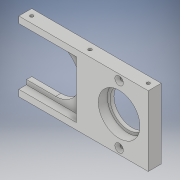
# Autodesk Inventor part: крепление подшипникового блока левая часть
Saved by Autodesk Inventor 2019.1 (Build 231200000, 200)
## iProperties
Created: 2018-08-01
Part Number: крепление подшипникового блока левая часть
Material: Типовые
Document SubType Name: Modeling
Designer: olege
Density: 1 g/cm^3
Appearance: По умолчанию
Author: olege
Autodesk Inventor part; units mm, degrees
ref_plane "YZ Plane" through (0, 0, 0) normal (1, 0, 0) x (0, 1, 0)
ref_plane "XZ Plane" through (0, 0, 0) normal (0, 1, 0) x (-1, 0, 0)
ref_plane "XY Plane" through (0, 0, 0) normal (0, 0, 1) x (1, 0, 0)
sketch "Эскиз1" plane through (0, 0, 0) normal (0, 0, 1) x (1, 0, 0)
  line L0 (50, -27) -> (-50, -27)
  line L1 (-50, -27) -> (-50, 27)
  line L2 (-50, 27) -> (50, 27)
  line L3 (50, 27) -> (50, -27)
  line L4 (50, -27) -> (-50, 27) construction
  line L5 (-50, -27) -> (50, 27) construction
  circle A0 centre (27.5, 0) radius 16.1
  point P0 (0, 0)
  point P1 (0, 0)
  dimension "d0" = 100
  dimension "d1" = 54
  dimension "d2" = 32.2
  dimension "d3" = 22.5
  constraints: 12 end point, 3 midpoint, 2 parallel, 1 centre point, 1 horizontal, 1 horizontal alignment, 1 perpendicular
  measures "d0" distance of L1.end L2.end
  measures "d1" distance of L0.end L1.end
  measures "d2" diameter of A0
  measures "d3" distance from line of L3 A0.centre
extrude "Выдавливание1" add sketch "Эскиз1" along normal blind 10
sketch "Эскиз2" plane through (0, 0, 0) normal (0, 0, -1) x (-1, 0, 0)
  circle A0 centre (-27.5, 0) radius 16.1 projected
  circle A1 centre (-27.5, 0) radius 14
  point P0 (0, 0)
  dimension "d6" = 28
  constraints: 1 centre point, 1 coincident
  measures "d6" diameter of A1
extrude "Выдавливание2" add sketch "Эскиз2" against normal blind 3
sketch "Эскиз3" plane through (0, 0, 10) normal (0, 0, 1) x (1, 0, 0)
  line L0 (-5.5, -22) -> (-5.5, 22) projected
  circle A0 centre (-27.5, 0) radius 18.5
  line L1 (-27.5, -18.5) -> (-62.6366, -18.5)
  line L2 (-62.6366, -18.5) -> (-62.6366, 18.5)
  line L3 (-62.6366, 18.5) -> (-27.5, 18.5)
  point P0 (0, 0)
  dimension "d9" = 37
  dimension "d10" = 22
  constraints: 6 end point, 2 perpendicular, 2 point on circle, 1 centre point, 1 horizontal, 1 horizontal alignment
  measures "d9" diameter of A0
  measures "d10" distance from line of L0 A0.centre
extrude "Выдавливание3" cut sketch "Эскиз3" against normal blind 28.4
sketch "Эскиз4" plane through (0, 0, 10) normal (0, 0, 1) x (1, 0, 0)
  line L0 (-5.5, -22) -> (-5.5, 22) projected
  line L1 (-51.5, 22) -> (-5.5, 22)
  line L2 (-5.5, 22) -> (-5.5, -22)
  line L3 (-5.5, -22) -> (-51.5, -22)
  line L4 (-51.5, -22) -> (-51.5, 22)
  line L5 (-51.5, 22) -> (-5.5, -22) construction
  line L6 (-5.5, 22) -> (-51.5, -22) construction
  point P0 (0, 0)
  point P1 (-28.5, 0)
  dimension "d13" = 46
  dimension "d14" = 44
  constraints: 12 end point, 2 midpoint, 2 parallel, 1 horizontal, 1 perpendicular
  measures "d13" distance of L0.start L3.end
  measures "d14" distance of L0.start L1.end
extrude "Выдавливание4" cut sketch "Эскиз4" against normal blind 6
sketch "Эскиз6" plane through (-50, 27, 0) normal (0, 1, 0) x (1, 0, 0)
  circle A0 centre (95, -5) radius 1.25
  circle A1 centre (50, -5) radius 1.25
  circle A2 centre (5, -5) radius 1.25
  line L0 (100, 0) -> (100, -10) projected
  line L1 (0, 0) -> (0, -10) projected
  line L2 (0, 0) -> (100, 0) projected
  point P0 (50, 0)
  point P1 (100, -5)
  point P2 (50, 0)
  dimension "d22" = 2.5
  dimension "d23" = 2.5
  dimension "d24" = 2.5
  dimension "d25" = 5
  dimension "d26" = 5
  constraints: 3 centre point, 3 horizontal alignment, 2 midpoint, 1 vertical alignment
  measures "d22" diameter of A0
  measures "d23" diameter of A1
  measures "d24" diameter of A2
  measures "d25" distance from line of L1 A2.centre
  measures "d26" distance of point (100, -5) A0.centre
extrude "Выдавливание6" cut sketch "Эскиз6" against normal up to surface (5 mm away)
sketch "Эскиз7" plane through (0, 0, 10) normal (0, 0, 1) x (1, 0, 0)
  circle A0 centre (27.5, 22.5) radius 1.25
  circle A1 centre (27.5, -22.5) radius 1.25
  circle A2 centre (27.5, 0) radius 16.1 projected
  point P0 (27.5, 0)
  dimension "d40" = 2.5
  dimension "d41" = 2.5
  dimension "d42" = 22.5
  dimension "d43" = 22.5
  constraints: 2 centre point, 2 vertical alignment, 1 coincident
  measures "d40" diameter of A0
  measures "d41" diameter of A1
  measures "d42" distance of A0.centre point (27.5, 0)
  measures "d43" distance of point (27.5, 0) A1.centre
extrude "Выдавливание7" cut sketch "Эскиз7" against normal blind 10 contours A0 | A1
chamfer "Фаска3" distance 2 angle 45 2 edges at (26.25, -22.5, 10) (26.25, 22.5, 10)
equation "\"d22\" = d23"
equation "\"d23\" = d24"
